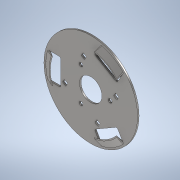
# Autodesk Inventor part: Tarcza_OsłonaA
Saved by Autodesk Inventor 2022 (Build 260153000, 153)
## iProperties
Created: 2021-06-26
Part Number: Tarcza_OsłonaA
Material: Stal, galwanizowana
Document SubType Name: Modeling
Designer: Matik
Density: 7.85 g/cm^3
Appearance: Galwanizowana
Author: Matik
Autodesk Inventor part; units mm, degrees
ref_plane "YZ Plane" through (0, 0, 0) normal (1, 0, 0) x (0, 1, 0)
ref_plane "XZ Plane" through (0, 0, 0) normal (0, 1, 0) x (-1, 0, 0)
ref_plane "Płaszczyzna konstrukcyjna1" through (0, 0, 0) normal (0, 0, 1) x (1, 0, 0)
sketch "Szkic1" plane through (0, 0, 0) normal (0, 0, 1) x (1, 0, 0)
  line L0 (-10.0657, 37.5657) -> (-5.7356, 35.0657) projected
  line L1 (-5.7356, 35.0657) -> (-8.2356, 30.7356) projected
  line L2 (-8.2356, 30.7356) -> (-12.5657, 33.2356) projected
  line L3 (-12.5657, 33.2356) -> (-10.0657, 37.5657) projected
  line L4 (-35.0657, -5.7356) -> (-30.7356, -8.2356) projected
  line L5 (-30.7356, -8.2356) -> (-33.2356, -12.5657) projected
  line L6 (-33.2356, -12.5657) -> (-37.5657, -10.0657) projected
  line L7 (-37.5657, -10.0657) -> (-35.0657, -5.7356) projected
  line L8 (8.2356, -30.7356) -> (12.5657, -33.2356) projected
  line L9 (12.5657, -33.2356) -> (10.0657, -37.5657) projected
  line L10 (10.0657, -37.5657) -> (5.7356, -35.0657) projected
  line L11 (5.7356, -35.0657) -> (8.2356, -30.7356) projected
  line L12 (33.2356, 12.5657) -> (37.5657, 10.0657) projected
  line L13 (37.5657, 10.0657) -> (35.0657, 5.7356) projected
  line L14 (35.0657, 5.7356) -> (30.7356, 8.2356) projected
  line L15 (30.7356, 8.2356) -> (33.2356, 12.5657) projected
  arc A0 (5.8446, 45.1231) -> (6.5766, 42.391) centre (7.5766, 44.1231) ccw projected
  line L16 (5.8446, 45.1231) -> (11.7077, 55.2784) projected
  arc A1 (13.6463, 56.2677) -> (11.7077, 55.2784) centre (13.4398, 54.2784) ccw projected
  arc A2 (41.9061, 39.9519) -> (13.6463, 56.2677) centre (9.5156, 16.4816) ccw projected
  arc A3 (42.0186, 37.7784) -> (41.9061, 39.9519) centre (40.2866, 38.7784) ccw projected
  line L17 (42.0186, 37.7784) -> (36.1554, 27.6231) projected
  arc A4 (33.4234, 26.891) -> (36.1554, 27.6231) centre (34.4234, 28.6231) ccw projected
  line L18 (33.4234, 26.891) -> (6.5766, 42.391) projected
  arc A5 (-53.7264, 17.5) -> (-55.5524, 16.3158) centre (-53.7264, 15.5) ccw projected
  line L19 (-53.7264, 17.5) -> (-42, 17.5) projected
  arc A6 (-40, 15.5) -> (-42, 17.5) centre (-42, 15.5) ccw projected
  line L20 (-40, 15.5) -> (-40, -15.5) projected
  arc A7 (-42, -17.5) -> (-40, -15.5) centre (-42, -15.5) ccw projected
  line L21 (-42, -17.5) -> (-53.7264, -17.5) projected
  arc A8 (-55.5524, -16.3158) -> (-53.7264, -17.5) centre (-53.7264, -15.5) ccw projected
  arc A9 (-55.5524, 16.3158) -> (-55.5524, -16.3158) centre (-19.0313, 0) ccw projected
  arc A10 (11.7077, -55.2784) -> (13.6463, -56.2677) centre (13.4398, -54.2784) ccw projected
  line L22 (11.7077, -55.2784) -> (5.8446, -45.1231) projected
  arc A11 (6.5766, -42.391) -> (5.8446, -45.1231) centre (7.5766, -44.1231) ccw projected
  line L23 (6.5766, -42.391) -> (33.4234, -26.891) projected
  arc A12 (36.1554, -27.6231) -> (33.4234, -26.891) centre (34.4234, -28.6231) ccw projected
  line L24 (36.1554, -27.6231) -> (42.0186, -37.7784) projected
  arc A13 (41.9061, -39.9519) -> (42.0186, -37.7784) centre (40.2866, -38.7784) ccw projected
  arc A14 (13.6463, -56.2677) -> (41.9061, -39.9519) centre (9.5156, -16.4816) ccw projected
  circle A15 centre (-13, 22.5167) radius 2.5 projected
  circle A16 centre (-13, -22.5167) radius 2.5 projected
  circle A17 centre (26, 0) radius 2.5 projected
  circle A18 centre (0, 0) radius 15 projected
  arc A19 (38.3351, 56.2857) -> (38.8994, 52.0753) centre (40.6782, 54.4567) ccw projected
  arc A20 (41.0855, 56.6743) -> (38.3351, 56.2857) centre (39.9117, 55.0551) ccw projected
  arc A21 (69.6301, 7.1871) -> (41.0855, 56.6743) centre (0, 0) ccw projected
  arc A22 (67.9165, 5.0008) -> (69.6301, 7.1871) centre (67.6406, 6.9817) ccw projected
  arc A23 (64.5545, 7.5974) -> (67.9165, 5.0008) centre (67.5065, 7.9448) ccw projected
  arc A24 (64.5545, 7.5974) -> (38.8994, 52.0753) centre (0, 0) ccw projected
  arc A25 (38.8568, -52.1071) -> (64.5482, -7.6502) centre (0, 0) ccw projected
  arc A26 (67.9124, -5.0563) -> (64.5482, -7.6502) centre (67.5, -8) ccw projected
  arc A27 (69.6242, -7.244) -> (67.9124, -5.0563) centre (67.6349, -7.037) ccw projected
  arc A28 (41.0392, -56.7079) -> (69.6242, -7.244) centre (0, 0) ccw projected
  arc A29 (38.2891, -56.317) -> (41.0392, -56.7079) centre (39.8667, -55.0877) ccw projected
  arc A30 (38.8568, -52.1071) -> (38.2891, -56.317) centre (40.6337, -54.4899) ccw projected
  arc A31 (-25.6977, -59.7045) -> (25.6489, -59.7255) centre (0, 0) ccw projected
  arc A32 (29.5773, -61.342) -> (25.6489, -59.7255) centre (26.8218, -62.4567) ccw projected
  arc A33 (28.5386, -63.9183) -> (29.5773, -61.342) centre (27.7232, -62.092) ccw projected
  arc A34 (-28.5909, -63.8949) -> (28.5386, -63.9183) centre (0, 0) ccw projected
  arc A35 (-29.6274, -61.3178) -> (-28.5909, -63.8949) centre (-27.774, -62.0694) ccw projected
  arc A36 (-25.6977, -59.7045) -> (-29.6274, -61.3178) centre (-26.8728, -62.4348) ccw projected
  arc A37 (-64.5545, -7.5974) -> (-38.8994, -52.0753) centre (0, 0) ccw projected
  arc A38 (-38.3351, -56.2857) -> (-38.8994, -52.0753) centre (-40.6782, -54.4567) ccw projected
  arc A39 (-41.0855, -56.6743) -> (-38.3351, -56.2857) centre (-39.9117, -55.0551) ccw projected
  arc A40 (-69.6301, -7.1871) -> (-41.0855, -56.6743) centre (0, 0) ccw projected
  arc A41 (-67.9165, -5.0008) -> (-69.6301, -7.1871) centre (-67.6406, -6.9817) ccw projected
  arc A42 (-64.5545, -7.5974) -> (-67.9165, -5.0008) centre (-67.5065, -7.9448) ccw projected
  arc A43 (-38.8568, 52.1071) -> (-64.5482, 7.6502) centre (0, 0) ccw projected
  arc A44 (-67.9124, 5.0563) -> (-64.5482, 7.6502) centre (-67.5, 8) ccw projected
  arc A45 (-69.6242, 7.244) -> (-67.9124, 5.0563) centre (-67.6349, 7.037) ccw projected
  arc A46 (-41.0392, 56.7079) -> (-69.6242, 7.244) centre (0, 0) ccw projected
  arc A47 (-38.2891, 56.317) -> (-41.0392, 56.7079) centre (-39.8667, 55.0877) ccw projected
  arc A48 (-38.8568, 52.1071) -> (-38.2891, 56.317) centre (-40.6337, 54.4899) ccw projected
  arc A49 (25.6977, 59.7045) -> (-25.6489, 59.7255) centre (0, 0) ccw projected
  arc A50 (-29.5773, 61.342) -> (-25.6489, 59.7255) centre (-26.8218, 62.4567) ccw projected
  arc A51 (-28.5386, 63.9183) -> (-29.5773, 61.342) centre (-27.7232, 62.092) ccw projected
  arc A52 (28.5909, 63.8949) -> (-28.5386, 63.9183) centre (0, 0) ccw projected
  arc A53 (29.6274, 61.3178) -> (28.5909, 63.8949) centre (27.774, 62.0694) ccw projected
  arc A54 (25.6977, 59.7045) -> (29.6274, 61.3178) centre (26.8728, 62.4348) ccw projected
  circle A55 centre (0, 0) radius 100 projected
  circle A56 centre (0, 0) radius 62.5
  point P0 (0, 0)
  dimension "d0" = 125
  constraints: 1 centre point, 1 coincident
  measures "d0" diameter of A56
extrude "Wyciągnięcie proste1" add sketch "Szkic1" along normal blind 2 contours A56
sketch "Szkic2" plane through (0, 0, 2) normal (0, 0, 1) x (1, 0, 0)
  arc A0 (15.0226, -58.0889) -> (42.7952, -42.0544) centre (0, 0) ccw
  arc A1 (13.6463, -56.2677) -> (41.9061, -39.9519) centre (9.5156, -16.4816) ccw projected
  arc A2 (11.7077, -55.2784) -> (13.6463, -56.2677) centre (13.4398, -54.2784) ccw projected
  arc A3 (41.9061, -39.9519) -> (42.0186, -37.7784) centre (40.2866, -38.7784) ccw projected
  line L0 (36.1554, -27.6231) -> (42.0186, -37.7784) projected
  line L1 (42.0186, -37.7784) -> (43.1007, -39.6526)
  line L2 (11.7077, -55.2784) -> (5.8446, -45.1231) projected
  line L3 (11.7077, -55.2784) -> (12.7898, -57.1526)
  arc A4 (42.7952, -42.0544) -> (43.1007, -39.6526) centre (41.3687, -40.6526) ccw
  arc A5 (12.7898, -57.1526) -> (15.0226, -58.0889) centre (14.5219, -56.1526) ccw
  point P0 (43.851, -40.9522)
  point P1 (13.5402, -58.4522)
  dimension "d3" = 120
  dimension "d4" = 2
  constraints: 8 point on circle, 6 tangent, 4 end point, 3 centre point, 2 point on line, 1 coincident, 1 collinear, 1 equal radius
  measures "d3" diameter of A0
  measures "d4" radius of A4
ref_plane "Płaszczyzna konstrukcyjna2" through (0, 0, 6) normal (0, 0, 1) x (1, 0, 0)
sketch "Szkic5" plane through (0, 0, 6) normal (0, 0, 1) x (1, 0, 0)
  arc A0 (8.9575, -49.1911) -> (38.1176, -32.3582) centre (0, 0) ccw
  arc A1 (9.7558, -50.5675) -> (38.9091, -33.7391) centre (0, 0) ccw
  line L0 (8.6959, -50.0777) -> (8.6118, -49.929)
  line L1 (11.7077, -55.2784) -> (5.8446, -45.1231) projected
  line L2 (36.1554, -27.6231) -> (42.0186, -37.7784) projected
  line L3 (39.0196, -32.584) -> (38.9317, -32.4318)
  arc A2 (8.6959, -50.0777) -> (9.7558, -50.5675) centre (9.5664, -49.5856) ccw
  arc A3 (8.9575, -49.1911) -> (8.6118, -49.929) centre (9.0471, -49.683) ccw
  arc A4 (38.9317, -32.4318) -> (38.1176, -32.3582) centre (38.4987, -32.6818) ccw
  arc A5 (38.9091, -33.7391) -> (39.0196, -32.584) centre (38.1536, -33.084) ccw
  point P0 (9.0471, -50.6991)
  point P1 (8.2633, -49.3125)
  point P2 (39.3732, -33.1964)
  point P3 (38.5742, -31.8125)
  dimension "d8" = 100
  dimension "d9" = 103
  dimension "d10" = 1
  dimension "d11" = 0.5
  dimension "d12" = 1
  constraints: 16 point on circle, 8 tangent, 7 point on line, 6 centre point, 4 end point, 2 coincident, 1 equal radius
  measures "d8" diameter of A0
  measures "d9" diameter of A1
  measures "d10" radius of A2
  measures "d11" radius of A3
  measures "d12" radius of A5
loft "Wyciągnięcie złożone1" add profiles "Szkic2", "Szkic5"
pattern_circular "Szyk kołowy1" count 3 over 360 about axis through (0, 0, 0) along (0, 0, 1) of "Wyciągnięcie złożone1"
